Autodesk Inventor part; units mm, degrees
(part 18 of 18)
sketch "Sketch18" plane through (0, 13.762, -7.5) normal (0, 1, 0) x (1, 0, 0)
  line L0 (-9.984, -8.484) -> (-9.984, 31.4609) projected
  line L1 (-9.984, 31.4609) -> (9.984, 31.4609) projected
  line L2 (9.984, 31.4609) -> (9.984, -8.484) projected
  line L3 (9.984, -8.484) -> (-9.984, -8.484) projected
  line L4 (11, -9.5) -> (11, 32.4769) projected
  line L5 (11, 32.4769) -> (-11, 32.4769) projected
  line L6 (-11, 32.4769) -> (-11, -9.5) projected
  line L7 (-11, -9.5) -> (11, -9.5) projected
  point P0 (0, -7.5)
  point P1 (-9.984, -7.5)
  point P2 (9.984, -7.5)
extrude "Extrusion13" add sketch "Sketch18" along normal blind 12 draft 6
sketch "Sketch19" plane through (0, 25.762, -7.5) normal (0, 1, 0) x (1, 0, 0)
  line L0 (-10.7373, 31.7382) -> (10.527, 31.7382)
  line L1 (10.527, 31.7382) -> (10.527, -9.2373)
  line L2 (10.527, -9.2373) -> (-10.7373, -9.2373)
  line L3 (-10.7373, -9.2373) -> (-10.7373, 31.7382)
  line L4 (-12.2613, 33.7382) -> (12.2613, 33.7382) projected
  line L5 (12.2613, -10.7613) -> (-12.2613, -10.7613) projected
  line L6 (-12.2613, -10.7613) -> (-12.2613, 33.7382) projected
  point P0 (0, -7.5)
  point P1 (-0.1051, 31.7382)
  point P2 (-0.1051, 30.8661)
  dimension "d183" = 2
  dimension "d184" = 1.524
  dimension "d185" = 1.524
  constraints: 8 end point, 2 parallel, 1 horizontal, 1 midpoint, 1 perpendicular, 1 vertical alignment
  measures "d183" distance between parallel lines of L0 L4
  measures "d184" distance between parallel lines of L5 L2
  measures "d185" distance between parallel lines of L3 L6
sketch "Sketch20" plane through (0, 13.762, -7.5) normal (0, 1, 0) x (-1, 0, 0)
  line L0 (9.984, 8.484) -> (-9.984, 8.484)
  line L1 (-9.984, 8.484) -> (-9.984, -31.4609)
  line L2 (-9.984, -31.4609) -> (9.984, -31.4609)
  line L3 (9.984, -31.4609) -> (9.984, 8.484)
  point P0 (0, 7.5)
  constraints: 8 end point, 2 parallel, 1 coincident, 1 horizontal, 1 perpendicular
loft "Loft1" cut profiles "Sketch20", "Sketch19"
ref_plane "Work Plane11" through (0, 0, -53) normal (0, 0, -1) x (-1, 0, 0)
sketch "Sketch29" plane through (2.8949, 25.762, -39.2382) normal (0, 0.9876883, 0.1564345) x (1, 0, 0)
  line L0 (-19.8442, 3.8517) -> (23.6634, 3.8517)
  line L1 (23.6634, 3.8517) -> (23.6634, -55.1626)
  line L2 (23.6634, -55.1626) -> (-19.8442, -55.1626)
  line L3 (-19.8442, -55.1626) -> (-19.8442, 3.8517)
  point P0 (0, 0)
  constraints: 8 end point, 2 parallel, 1 horizontal, 1 perpendicular
extrude "Extrusion16" cut sketch "Sketch29" along normal through all
sketch "Sketch31" plane through (2.8949, 25.762, -39.2382) normal (0, 0.9876883, 0.1564345) x (1, 0, 0)
  line L0 (8.6705, -42.3246) -> (-14.4602, -42.3246) projected
  line L1 (-14.4602, -42.3246) -> (-15.1561, 0) projected
  line L2 (-13.7107, 0.9594) -> (7.7107, 0.9594)
  line L3 (7.7107, 0.9594) -> (7.7107, -41.5626)
  line L4 (7.7107, -41.5626) -> (-13.7107, -41.5626)
  line L5 (-13.7107, -41.5626) -> (-13.7107, 0.9594)
  line L6 (-2.8949, 132.5532) -> (-2.8949, -156.9203) projected
  line L7 (-13.6321, 0) -> (7.6321, 0) projected
  line L8 (-15.1561, 1.9754) -> (9.3664, 1.9754) projected
  point P0 (-2.8949, -42.7851)
  point P1 (-3, 0.9594)
  point P2 (-3, 0)
  point P3 (-14.3631, -48.2313)
  dimension "d198" = 1.016
  dimension "d199" = 0.762
  dimension "d200" = 0.762
  constraints: 8 end point, 2 midpoint, 2 parallel, 1 horizontal, 1 perpendicular, 1 vertical alignment
  measures "d198" distance between parallel lines of L2 L8
  measures "d199" distance between parallel lines of L0 L4
  measures "d200" distance from line of L4.end L1
extrude "Extrusion18" cut sketch "Sketch31" against normal blind 0.508
sketch "Sketch38" plane through (0, 13.762, -7.5) normal (0, 1, 0) x (-1, 0, 0)
  line L0 (-9.984, 8.484) -> (9.984, 8.484) projected
  line L1 (-11, 9.5) -> (-11.5654, 10.0654) projected
  line L2 (11, 9.5) -> (-11, 9.5) projected
  line L3 (11, -32.4769) -> (11, 9.5) projected
  line L4 (-11, 9.5) -> (-11, -32.4769) projected
  line L5 (0, -149.2871) -> (0, 99.3442) projected
  arc A0 (10.8101, 9.5) -> (-11, 9.5) centre (-0.0949, 6.068) ccw
  line L6 (-11, 9.5) -> (11, 9.5)
  point P0 (0, 7.5)
  point P1 (0, 17.5)
  point P2 (0, 9.5)
  dimension "d218" = 8
  constraints: 3 point on circle, 2 end point, 2 point on line, 1 centre point, 1 midpoint, 1 perpendicular
  measures "d218" distance of point (0, 9.5) point (0, 17.5)
extrude "Extrusion20" add sketch "Sketch38" against normal up to next
sketch "Sketch39" plane through (2.8949, 25.762, -39.2382) normal (0, 0.9876883, 0.1564345) x (1, 0, 0)
  line L0 (-2.8949, 132.5532) -> (-2.8949, -156.9203) projected
  arc A0 (-14.4602, -42.3246) -> (8.6705, -42.3246) centre (-2.8949, -19.2749) ccw
  line L1 (-14.4602, -42.3246) -> (8.6705, -42.3246)
  point P0 (-2.8949, -42.7851)
  constraints: 2 end point, 2 point on circle, 1 centre point, 1 perpendicular
loft "Loft6" add profiles "Sketch39" section 2 edges at (0.0949, 13.762, 2) (0.0949, 13.762, 10.0004)
equation "\"d22\" = d24"
equation "\"d23\" = d24"
equation "\"d37\" = t"
equation "\"d40\" = t"
equation "\"t\" = 1.016"
equation "\"d14\" = d24"
equation "\"d24\" = 1.016"
body "Solid1"
